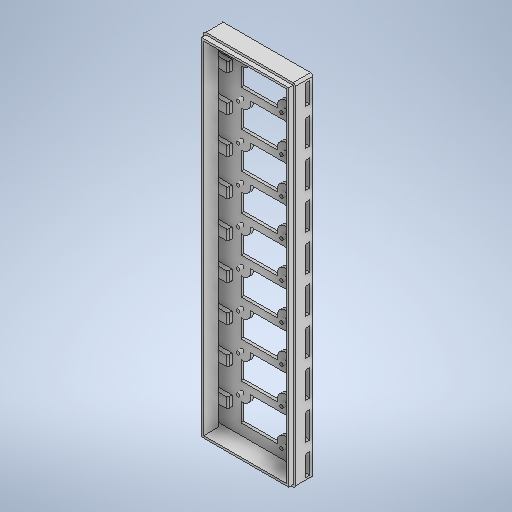
# Autodesk Inventor part: lm2596_socket
Saved by Autodesk Inventor 2025 (Build 290162000, 162)
## iProperties
Created: 2025-01-25
Part Number: lm2596_socket
Material: Všeobecné
Document SubType Name: Modeling
Designer: lukas
Density: 1 g/cm^3
Appearance: Výchozí
Author: lukas
## iProperties of the stored document lm2596_socket_3D tisk.ipt
Created: 2025-01-25
Part Number: lm2596_socket_3D tisk
Material: Všeobecné
Document SubType Name: Modeling
Designer: lukas
Density: 1 g/cm^3
Appearance: Výchozí
Author: lukas
Autodesk Inventor part; units mm, degrees
ref_plane "YZ Plane" through (0, 0, 0) normal (1, 0, 0) x (0, 1, 0)
ref_plane "XZ Plane" through (0, 0, 0) normal (0, 1, 0) x (-1, 0, 0)
ref_plane "XY Plane" through (0, 0, 0) normal (0, 0, 1) x (1, 0, 0)
sketch "Náčrt1" plane through (0, 0, 0) normal (0, 0, 1) x (1, 0, 0)
  line L0 (0, 17.5) -> (0, -17.5) projected
  line L1 (-32.9, 0) -> (32.9, 0) projected
  line L2 (23.5, -12.5) -> (-23.5, -12.5)
  line L3 (-23.5, -12.5) -> (-23.5, 12.5)
  line L4 (-23.5, 12.5) -> (23.5, 12.5)
  line L5 (23.5, 12.5) -> (23.5, -12.5)
  point P0 (0, 0)
  dimension "d0" = 47
  dimension "d1" = 25
  constraints: 8 end point, 2 parallel, 1 horizontal, 1 perpendicular, 2 other
  measures "d0" distance between parallel lines of L3 L5
  measures "d1" distance between parallel lines of L4 L2
extrude "Vysunutí1" add sketch "Náčrt1" along normal blind 2
sketch "Náčrt2" plane through (0, 0, 2) normal (0, 0, 1) x (1, 0, 0)
  line L0 (23.5, 12.5) -> (-23.5, 12.5) projected
  line L1 (-23.5, 12.5) -> (-23.5, -12.5) projected
  line L2 (-23.5, -12.5) -> (23.5, -12.5) projected
  line L3 (23.5, -12.5) -> (23.5, 12.5) projected
  line L4 (0, 17.5) -> (0, -17.5) projected
  line L5 (-32.9, 0) -> (32.9, 0) projected
  circle A0 centre (-15, 8.5) radius 1.2
  circle A1 centre (15, -8.5) radius 1.2
  point P0 (0, 0)
  dimension "d4" = 2.4
  dimension "d5" = 4
  dimension "d9" = 180
  dimension "d18" = 8.5
  constraints: 2 centre point, 3 other
  measures "d4" diameter of A0
  measures "d5" distance from line of A0.centre L0
  measures "d18" distance from line of L1 A0.centre
extrude "Vysunutí2" add sketch "Náčrt2" along normal blind 3 contours A0 | A1
sketch "Náčrt3" plane through (0, 0, 2) normal (0, 0, 1) x (1, 0, 0)
  circle A0 centre (15, -8.5) radius 1.2 projected
  circle A1 centre (-15, 8.5) radius 1.2 projected
  line L0 (23.5, 12.5) -> (-23.5, 12.5) projected
  line L1 (-23.5, 12.5) -> (-23.5, -12.5) projected
  line L2 (-23.5, -12.5) -> (23.5, -12.5) projected
  line L3 (23.5, -12.5) -> (23.5, 12.5) projected
  line L4 (0, 17.5) -> (0, -17.5) projected
  line L5 (-32.9, 0) -> (32.9, 0) projected
  line L6 (-23.5, 12.5) -> (-23.5, -12.5) projected
  line L7 (-22, -3.5) -> (-23.5, -3.5)
  line L8 (-23.5, -3.5) -> (-23.5, 3.5)
  line L9 (-23.5, 3.5) -> (-22, 3.5)
  line L10 (-22, 3.5) -> (-22, -3.5)
  line L11 (23.5, -3.5) -> (22, -3.5)
  line L12 (22, -3.5) -> (22, 3.5)
  line L13 (22, 3.5) -> (23.5, 3.5)
  line L14 (23.5, 3.5) -> (23.5, -3.5)
  line L15 (22, -3.5) -> (23.5, -3.5)
  line L16 (23.5, -3.5) -> (23.5, 0)
  line L17 (23.5, 0) -> (22, 0)
  line L18 (22, 0) -> (22, -3.5)
  line L19 (-22, -3.5) -> (-23.5, -3.5)
  line L20 (-23.5, -3.5) -> (-23.5, 0)
  line L21 (-23.5, 0) -> (-22, 0)
  line L22 (-22, 0) -> (-22, -3.5)
  point P0 (0, 0)
  point P1 (22, 0)
  point P2 (-22, 0)
  point P3 (-23.5, 3.5)
  point P4 (-23.5, -3.5)
  dimension "d13" = 7
  dimension "d14" = 7
  dimension "d15" = 44
  constraints: 32 end point, 8 parallel, 4 horizontal, 4 perpendicular, 2 midpoint, 2 point on line, 3 other
  measures "d13" distance of L9.end L7.start
  measures "d14" distance of L11.end L12.end
  measures "d15" distance between parallel lines of L10 L12
extrude "Vysunutí3" add sketch "Náčrt3" along normal blind 3 contours L3 L5 L12 L13 | L3 L11 L12 L5 | L9 L10 L5 L1 | L10 L7 L1 L5
sketch "Náčrt4" plane through (0, 0, 2) normal (0, 0, 1) x (1, 0, 0)
  line L0 (22, 3.5) -> (23.5, 3.5) projected
  line L1 (23.5, 3.5) -> (23.5, 12.5) projected
  line L2 (23.5, 12.5) -> (-23.5, 12.5) projected
  line L3 (-23.5, 12.5) -> (-23.5, 3.5) projected
  line L4 (-23.5, 3.5) -> (-22, 3.5) projected
  line L5 (-22, 3.5) -> (-22, -3.5) projected
  line L6 (-22, -3.5) -> (-23.5, -3.5) projected
  line L7 (-23.5, -3.5) -> (-23.5, -12.5) projected
  line L8 (-23.5, -12.5) -> (23.5, -12.5) projected
  line L9 (23.5, -12.5) -> (23.5, -3.5) projected
  line L10 (23.5, -3.5) -> (22, -3.5) projected
  line L11 (22, -3.5) -> (22, 3.5) projected
  circle A0 centre (15, -8.5) radius 1.2 projected
  circle A1 centre (-15, 8.5) radius 1.2 projected
  line L12 (15.8095, 10) -> (15.8095, -2.5549)
  line L13 (-15.8095, -10) -> (-15.8095, 2.5549)
  line L14 (0, 17.5) -> (0, -17.5) projected
  line L15 (-32.9, 0) -> (32.9, 0) projected
  arc A2 (-15.8095, 2.5549) -> (-9.1905, 10) centre (-15, 8.5) ccw
  arc A3 (15.8095, -2.5549) -> (9.1905, -10) centre (15, -8.5) ccw
  line L16 (-9.1905, 10) -> (15.8095, 10)
  line L17 (9.1905, -10) -> (-15.8095, -10)
  point P0 (0, 0)
  dimension "d21" = 12
  dimension "d22" = 12
  dimension "d23" = 20
  dimension "d25" = 25
  dimension "d26" = 25
  constraints: 8 end point, 4 point on circle, 2 centre point, 2 coincident, 2 parallel, 1 horizontal, 1 perpendicular, 1 other
  measures "d21" diameter of A2
  measures "d22" diameter of A3
  measures "d23" distance between parallel lines of L16 L17
  measures "d25" distance of L16.start L12.start
  measures "d26" distance of L17.start L13.start
extrude "Vysunutí4" cut sketch "Náčrt4" against normal through all contours L15 L14 L16 L12 | L12 A3 L17 L14 L15 | L15 L13 A2 L16 L14 | L14 L17 L13 L15
pattern_linear "Obdélníkové pole1" count 9 spacing 25 along (0, 1, 0) first direction both ways yes
sketch "Náčrt5" plane through (0, 0, 0) normal (0, 0, 1) x (1, 0, 0)
  line L0 (-15.8095, 15) -> (9.1905, 15) projected
  arc A0 (15.8095, 22.4451) -> (9.1905, 15) centre (15, 16.5) ccw projected
  line L1 (15.8095, 22.4451) -> (15.8095, 35) projected
  line L2 (15.8095, 35) -> (-9.1905, 35) projected
  arc A1 (-15.8095, 27.5549) -> (-9.1905, 35) centre (-15, 33.5) ccw projected
  line L3 (-15.8095, 27.5549) -> (-15.8095, 15) projected
  line L4 (-15.8095, 40) -> (9.1905, 40) projected
  arc A2 (15.8095, 47.4451) -> (9.1905, 40) centre (15, 41.5) ccw projected
  line L5 (15.8095, 47.4451) -> (15.8095, 60) projected
  line L6 (15.8095, 60) -> (-9.1905, 60) projected
  arc A3 (-15.8095, 52.5549) -> (-9.1905, 60) centre (-15, 58.5) ccw projected
  line L7 (-15.8095, 52.5549) -> (-15.8095, 40) projected
  line L8 (-15.8095, 65) -> (9.1905, 65) projected
  arc A4 (15.8095, 72.4451) -> (9.1905, 65) centre (15, 66.5) ccw projected
  line L9 (15.8095, 72.4451) -> (15.8095, 85) projected
  line L10 (15.8095, 85) -> (-9.1905, 85) projected
  arc A5 (-15.8095, 77.5549) -> (-9.1905, 85) centre (-15, 83.5) ccw projected
  line L11 (-15.8095, 77.5549) -> (-15.8095, 65) projected
  line L12 (-15.8095, 90) -> (9.1905, 90) projected
  arc A6 (15.8095, 97.4451) -> (9.1905, 90) centre (15, 91.5) ccw projected
  line L13 (15.8095, 97.4451) -> (15.8095, 110) projected
  line L14 (15.8095, 110) -> (-9.1905, 110) projected
  arc A7 (-15.8095, 102.5549) -> (-9.1905, 110) centre (-15, 108.5) ccw projected
  line L15 (-15.8095, 102.5549) -> (-15.8095, 90) projected
  line L16 (-15.8095, -110) -> (9.1905, -110) projected
  arc A8 (15.8095, -102.5549) -> (9.1905, -110) centre (15, -108.5) ccw projected
  line L17 (15.8095, -102.5549) -> (15.8095, -90) projected
  line L18 (15.8095, -90) -> (-9.1905, -90) projected
  arc A9 (-15.8095, -97.4451) -> (-9.1905, -90) centre (-15, -91.5) ccw projected
  line L19 (-15.8095, -97.4451) -> (-15.8095, -110) projected
  line L20 (-15.8095, -85) -> (9.1905, -85) projected
  arc A10 (15.8095, -77.5549) -> (9.1905, -85) centre (15, -83.5) ccw projected
  line L21 (15.8095, -77.5549) -> (15.8095, -65) projected
  line L22 (15.8095, -65) -> (-9.1905, -65) projected
  arc A11 (-15.8095, -72.4451) -> (-9.1905, -65) centre (-15, -66.5) ccw projected
  line L23 (-15.8095, -72.4451) -> (-15.8095, -85) projected
  line L24 (-15.8095, -60) -> (9.1905, -60) projected
  arc A12 (15.8095, -52.5549) -> (9.1905, -60) centre (15, -58.5) ccw projected
  line L25 (15.8095, -52.5549) -> (15.8095, -40) projected
  line L26 (15.8095, -40) -> (-9.1905, -40) projected
  arc A13 (-15.8095, -47.4451) -> (-9.1905, -40) centre (-15, -41.5) ccw projected
  line L27 (-15.8095, -47.4451) -> (-15.8095, -60) projected
  line L28 (-15.8095, -35) -> (9.1905, -35) projected
  arc A14 (15.8095, -27.5549) -> (9.1905, -35) centre (15, -33.5) ccw projected
  line L29 (15.8095, -27.5549) -> (15.8095, -15) projected
  line L30 (15.8095, -15) -> (-9.1905, -15) projected
  arc A15 (-15.8095, -22.4451) -> (-9.1905, -15) centre (-15, -16.5) ccw projected
  line L31 (-15.8095, -22.4451) -> (-15.8095, -35) projected
  line L32 (-15.8095, -10) -> (9.1905, -10) projected
  arc A16 (15.8095, -2.5549) -> (9.1905, -10) centre (15, -8.5) ccw projected
  line L33 (15.8095, -2.5549) -> (15.8095, 10) projected
  line L34 (15.8095, 10) -> (-9.1905, 10) projected
  arc A17 (-15.8095, 2.5549) -> (-9.1905, 10) centre (-15, 8.5) ccw projected
  line L35 (-15.8095, 2.5549) -> (-15.8095, -10) projected
  line L36 (23.5, -112.5) -> (23.5, 112.5) projected
  line L37 (-23.5, -112.5) -> (23.5, -112.5) projected
  line L38 (-23.5, 112.5) -> (-23.5, -112.5) projected
  line L39 (23.5, 112.5) -> (-23.5, 112.5) projected
  line L40 (31.5, 120.5) -> (31.5, -120.5)
  line L41 (31.5, -120.5) -> (-31.5, -120.5)
  line L42 (-31.5, -120.5) -> (-31.5, 120.5)
  line L43 (-31.5, 120.5) -> (31.5, 120.5)
  line L44 (23.5, 112.5) -> (-23.5, 112.5)
  line L45 (-23.5, 112.5) -> (-23.5, -112.5)
  line L46 (-23.5, -112.5) -> (23.5, -112.5)
  line L47 (23.5, -112.5) -> (23.5, 112.5)
  point P0 (0, 0)
  dimension "d33" = 8
  constraints: 16 end point, 2 parallel, 1 horizontal, 1 perpendicular, 3 other
  measures "d33" distance between parallel lines of L36 L40
extrude "Vysunutí5" add sketch "Náčrt5" along normal blind 2 contours L40 L41 L42 L43
sketch "Náčrt6" plane through (0, 0, 2) normal (0, 0, 1) x (1, 0, 0)
  line L0 (-23.5, -21.5) -> (-22, -21.5) projected
  line L1 (-22, -21.5) -> (-22, -28.5) projected
  line L2 (-22, -28.5) -> (-23.5, -28.5) projected
  line L3 (-23.5, -21.5) -> (-23.5, -28.5) projected
  line L4 (-23.5, -46.5) -> (-22, -46.5) projected
  line L5 (-22, -46.5) -> (-22, -53.5) projected
  line L6 (-22, -53.5) -> (-23.5, -53.5) projected
  line L7 (-23.5, -46.5) -> (-23.5, -53.5) projected
  line L8 (-23.5, 3.5) -> (-23.5, -3.5) projected
  line L9 (-23.5, 3.5) -> (-22, 3.5) projected
  line L10 (-22, 3.5) -> (-22, -3.5) projected
  line L11 (-22, -3.5) -> (-23.5, -3.5) projected
  line L12 (-23.5, -71.5) -> (-22, -71.5) projected
  line L13 (-22, -71.5) -> (-22, -78.5) projected
  line L14 (-22, -78.5) -> (-23.5, -78.5) projected
  line L15 (-23.5, -71.5) -> (-23.5, -78.5) projected
  line L16 (23.5, -28.5) -> (22, -28.5) projected
  line L17 (22, -28.5) -> (22, -21.5) projected
  line L18 (22, -21.5) -> (23.5, -21.5) projected
  line L19 (23.5, -28.5) -> (23.5, -21.5) projected
  line L20 (23.5, -53.5) -> (23.5, -46.5) projected
  line L21 (23.5, -53.5) -> (22, -53.5) projected
  line L22 (22, -53.5) -> (22, -46.5) projected
  line L23 (22, -46.5) -> (23.5, -46.5) projected
  line L24 (-23.5, 28.5) -> (-23.5, 21.5) projected
  line L25 (-23.5, 28.5) -> (-22, 28.5) projected
  line L26 (-22, 28.5) -> (-22, 21.5) projected
  line L27 (-22, 21.5) -> (-23.5, 21.5) projected
  line L28 (-23.5, -96.5) -> (-22, -96.5) projected
  line L29 (-22, -96.5) -> (-22, -103.5) projected
  line L30 (-22, -103.5) -> (-23.5, -103.5) projected
  line L31 (-23.5, -96.5) -> (-23.5, -103.5) projected
  line L32 (23.5, -3.5) -> (22, -3.5) projected
  line L33 (22, -3.5) -> (22, 3.5) projected
  line L34 (22, 3.5) -> (23.5, 3.5) projected
  line L35 (23.5, -3.5) -> (23.5, 3.5) projected
  line L36 (23.5, -78.5) -> (23.5, -71.5) projected
  line L37 (23.5, -78.5) -> (22, -78.5) projected
  line L38 (22, -78.5) -> (22, -71.5) projected
  line L39 (22, -71.5) -> (23.5, -71.5) projected
  line L40 (-23.5, 53.5) -> (-23.5, 46.5) projected
  line L41 (-23.5, 53.5) -> (-22, 53.5) projected
  line L42 (-22, 53.5) -> (-22, 46.5) projected
  line L43 (-22, 46.5) -> (-23.5, 46.5) projected
  line L44 (23.5, 21.5) -> (22, 21.5) projected
  line L45 (22, 21.5) -> (22, 28.5) projected
  line L46 (22, 28.5) -> (23.5, 28.5) projected
  line L47 (23.5, 21.5) -> (23.5, 28.5) projected
  line L48 (23.5, -103.5) -> (23.5, -96.5) projected
  line L49 (23.5, -103.5) -> (22, -103.5) projected
  line L50 (22, -103.5) -> (22, -96.5) projected
  line L51 (22, -96.5) -> (23.5, -96.5) projected
  line L52 (-23.5, 78.5) -> (-23.5, 71.5) projected
  line L53 (-23.5, 78.5) -> (-22, 78.5) projected
  line L54 (-22, 78.5) -> (-22, 71.5) projected
  line L55 (-22, 71.5) -> (-23.5, 71.5) projected
  line L56 (23.5, 46.5) -> (22, 46.5) projected
  line L57 (22, 46.5) -> (22, 53.5) projected
  line L58 (22, 53.5) -> (23.5, 53.5) projected
  line L59 (23.5, 46.5) -> (23.5, 53.5) projected
  line L60 (23.5, 71.5) -> (22, 71.5) projected
  line L61 (22, 71.5) -> (22, 78.5) projected
  line L62 (22, 78.5) -> (23.5, 78.5) projected
  line L63 (23.5, 71.5) -> (23.5, 78.5) projected
  line L64 (-23.5, 103.5) -> (-23.5, 96.5) projected
  line L65 (-23.5, 103.5) -> (-22, 103.5) projected
  line L66 (-22, 103.5) -> (-22, 96.5) projected
  line L67 (-22, 96.5) -> (-23.5, 96.5) projected
  line L68 (-31.5, 120.5) -> (-31.5, -120.5) projected
  line L69 (-31.5, -120.5) -> (31.5, -120.5) projected
  line L70 (31.5, -120.5) -> (31.5, 120.5) projected
  line L71 (31.5, 120.5) -> (-31.5, 120.5) projected
  circle A0 centre (-15, 33.5) radius 1.2 projected
  circle A1 centre (15, 16.5) radius 1.2 projected
  line L72 (9.1905, 15) -> (-15.8095, 15) projected
  line L73 (-15.8095, 15) -> (-15.8095, 27.5549) projected
  arc A2 (-15.8095, 27.5549) -> (-9.1905, 35) centre (-15, 33.5) ccw projected
  line L74 (-9.1905, 35) -> (15.8095, 35) projected
  line L75 (15.8095, 35) -> (15.8095, 22.4451) projected
  arc A3 (15.8095, 22.4451) -> (9.1905, 15) centre (15, 16.5) ccw projected
  line L76 (9.1905, 40) -> (-15.8095, 40) projected
  line L77 (-15.8095, 40) -> (-15.8095, 52.5549) projected
  arc A4 (-15.8095, 52.5549) -> (-9.1905, 60) centre (-15, 58.5) ccw projected
  line L78 (-9.1905, 60) -> (15.8095, 60) projected
  line L79 (15.8095, 60) -> (15.8095, 47.4451) projected
  arc A5 (15.8095, 47.4451) -> (9.1905, 40) centre (15, 41.5) ccw projected
  circle A6 centre (15, 41.5) radius 1.2 projected
  circle A7 centre (-15, 58.5) radius 1.2 projected
  line L80 (9.1905, 65) -> (-15.8095, 65) projected
  line L81 (-15.8095, 65) -> (-15.8095, 77.5549) projected
  arc A8 (-15.8095, 77.5549) -> (-9.1905, 85) centre (-15, 83.5) ccw projected
  line L82 (-9.1905, 85) -> (15.8095, 85) projected
  line L83 (15.8095, 85) -> (15.8095, 72.4451) projected
  arc A9 (15.8095, 72.4451) -> (9.1905, 65) centre (15, 66.5) ccw projected
  circle A10 centre (15, 66.5) radius 1.2 projected
  circle A11 centre (-15, 83.5) radius 1.2 projected
  line L84 (9.1905, 90) -> (-15.8095, 90) projected
  line L85 (-15.8095, 90) -> (-15.8095, 102.5549) projected
  arc A12 (-15.8095, 102.5549) -> (-9.1905, 110) centre (-15, 108.5) ccw projected
  line L86 (-9.1905, 110) -> (15.8095, 110) projected
  line L87 (15.8095, 110) -> (15.8095, 97.4451) projected
  arc A13 (15.8095, 97.4451) -> (9.1905, 90) centre (15, 91.5) ccw projected
  circle A14 centre (15, 91.5) radius 1.2 projected
  circle A15 centre (-15, 108.5) radius 1.2 projected
  circle A16 centre (-15, -91.5) radius 1.2 projected
  circle A17 centre (15, -108.5) radius 1.2 projected
  line L88 (9.1905, -110) -> (-15.8095, -110) projected
  line L89 (-15.8095, -110) -> (-15.8095, -97.4451) projected
  arc A18 (-15.8095, -97.4451) -> (-9.1905, -90) centre (-15, -91.5) ccw projected
  line L90 (-9.1905, -90) -> (15.8095, -90) projected
  line L91 (15.8095, -90) -> (15.8095, -102.5549) projected
  arc A19 (15.8095, -102.5549) -> (9.1905, -110) centre (15, -108.5) ccw projected
  line L92 (9.1905, -85) -> (-15.8095, -85) projected
  line L93 (-15.8095, -85) -> (-15.8095, -72.4451) projected
  arc A20 (-15.8095, -72.4451) -> (-9.1905, -65) centre (-15, -66.5) ccw projected
  line L94 (-9.1905, -65) -> (15.8095, -65) projected
  line L95 (15.8095, -65) -> (15.8095, -77.5549) projected
  arc A21 (15.8095, -77.5549) -> (9.1905, -85) centre (15, -83.5) ccw projected
  circle A22 centre (15, -83.5) radius 1.2 projected
  circle A23 centre (-15, -66.5) radius 1.2 projected
  line L96 (9.1905, -60) -> (-15.8095, -60) projected
  line L97 (-15.8095, -60) -> (-15.8095, -47.4451) projected
  arc A24 (-15.8095, -47.4451) -> (-9.1905, -40) centre (-15, -41.5) ccw projected
  line L98 (-9.1905, -40) -> (15.8095, -40) projected
  line L99 (15.8095, -40) -> (15.8095, -52.5549) projected
  arc A25 (15.8095, -52.5549) -> (9.1905, -60) centre (15, -58.5) ccw projected
  circle A26 centre (15, -58.5) radius 1.2 projected
  circle A27 centre (-15, -41.5) radius 1.2 projected
  line L100 (9.1905, -35) -> (-15.8095, -35) projected
  line L101 (-15.8095, -35) -> (-15.8095, -22.4451) projected
  arc A28 (-15.8095, -22.4451) -> (-9.1905, -15) centre (-15, -16.5) ccw projected
  line L102 (-9.1905, -15) -> (15.8095, -15) projected
  line L103 (15.8095, -15) -> (15.8095, -27.5549) projected
  arc A29 (15.8095, -27.5549) -> (9.1905, -35) centre (15, -33.5) ccw projected
  circle A30 centre (15, -33.5) radius 1.2 projected
  circle A31 centre (-15, -16.5) radius 1.2 projected
  line L104 (9.1905, -10) -> (-15.8095, -10) projected
  line L105 (-15.8095, -10) -> (-15.8095, 2.5549) projected
  arc A32 (-15.8095, 2.5549) -> (-9.1905, 10) centre (-15, 8.5) ccw projected
  line L106 (-9.1905, 10) -> (15.8095, 10) projected
  line L107 (15.8095, 10) -> (15.8095, -2.5549) projected
  arc A33 (15.8095, -2.5549) -> (9.1905, -10) centre (15, -8.5) ccw projected
  line L108 (23.5, 96.5) -> (23.5, 103.5) projected
  line L109 (23.5, 96.5) -> (22, 96.5) projected
  line L110 (22, 96.5) -> (22, 103.5) projected
  line L111 (22, 103.5) -> (23.5, 103.5) projected
  circle A34 centre (15, -8.5) radius 1.2 projected
  circle A35 centre (-15, 8.5) radius 1.2 projected
  line L112 (28.5, 117.5) -> (28.5, -117.5)
  line L113 (28.5, -117.5) -> (-28.5, -117.5)
  line L114 (-28.5, -117.5) -> (-28.5, 117.5)
  line L115 (-28.5, 117.5) -> (28.5, 117.5)
  line L116 (31.5, 120.5) -> (-31.5, 120.5)
  line L117 (-31.5, 120.5) -> (-31.5, -120.5)
  line L118 (-31.5, -120.5) -> (31.5, -120.5)
  line L119 (31.5, -120.5) -> (31.5, 120.5)
  point P0 (0, 0)
  dimension "d36" = 3
  constraints: 16 end point, 2 parallel, 1 horizontal, 1 perpendicular, 3 other
  measures "d36" distance between parallel lines of L70 L112
extrude "Vysunutí6" add sketch "Náčrt6" along normal blind 10 contours L71 L70 L69 L68
sketch "Náčrt7" plane through (-31.5, -120.5, 0) normal (-1, 0, 0) x (0, 0, 1)
  line L0 (0, 289.2) -> (0, -48.2) projected
  line L1 (-2.4, 120.5) -> (14.4, 120.5) projected
  line L2 (2, 238) -> (2, 3) projected
  line L3 (2, 3) -> (2, 238) projected
  line L4 (2, 99) -> (2, 92) projected
  line L5 (2, 99) -> (2, 92) projected
  line L6 (2, 74) -> (2, 67) projected
  line L7 (2, 74) -> (2, 67) projected
  line L8 (2, 124) -> (2, 117) projected
  line L9 (2, 124) -> (2, 117) projected
  line L10 (2, 49) -> (2, 42) projected
  line L11 (2, 49) -> (2, 42) projected
  line L12 (2, 92) -> (2, 99) projected
  line L13 (2, 92) -> (2, 99) projected
  line L14 (2, 67) -> (2, 74) projected
  line L15 (2, 67) -> (2, 74) projected
  line L16 (2, 149) -> (2, 142) projected
  line L17 (2, 149) -> (2, 142) projected
  line L18 (2, 24) -> (2, 17) projected
  line L19 (2, 24) -> (2, 17) projected
  line L20 (2, 117) -> (2, 124) projected
  line L21 (2, 117) -> (2, 124) projected
  line L22 (2, 42) -> (2, 49) projected
  line L23 (2, 42) -> (2, 49) projected
  line L24 (2, 174) -> (2, 167) projected
  line L25 (2, 174) -> (2, 167) projected
  line L26 (2, 142) -> (2, 149) projected
  line L27 (2, 142) -> (2, 149) projected
  line L28 (2, 17) -> (2, 24) projected
  line L29 (2, 17) -> (2, 24) projected
  line L30 (2, 199) -> (2, 192) projected
  line L31 (2, 199) -> (2, 192) projected
  line L32 (2, 167) -> (2, 174) projected
  line L33 (2, 167) -> (2, 174) projected
  line L34 (2, 192) -> (2, 199) projected
  line L35 (2, 192) -> (2, 199) projected
  line L36 (2, 224) -> (2, 217) projected
  line L37 (2, 224) -> (2, 217) projected
  line L38 (2, 155.2) -> (2, 152.8) projected
  line L39 (2, 138.2) -> (2, 135.8) projected
  line L40 (2, 135.5) -> (2, 148.0549) projected
  line L41 (2, 148.0549) -> (2, 155.5) projected
  line L42 (2, 155.5) -> (2, 142.9451) projected
  line L43 (2, 142.9451) -> (2, 135.5) projected
  line L44 (2, 160.5) -> (2, 173.0549) projected
  line L45 (2, 173.0549) -> (2, 180.5) projected
  line L46 (2, 180.5) -> (2, 167.9451) projected
  line L47 (2, 167.9451) -> (2, 160.5) projected
  line L48 (2, 163.2) -> (2, 160.8) projected
  line L49 (2, 180.2) -> (2, 177.8) projected
  line L50 (2, 185.5) -> (2, 198.0549) projected
  line L51 (2, 198.0549) -> (2, 205.5) projected
  line L52 (2, 205.5) -> (2, 192.9451) projected
  line L53 (2, 192.9451) -> (2, 185.5) projected
  line L54 (2, 188.2) -> (2, 185.8) projected
  line L55 (2, 205.2) -> (2, 202.8) projected
  line L56 (2, 210.5) -> (2, 223.0549) projected
  line L57 (2, 223.0549) -> (2, 230.5) projected
  line L58 (2, 230.5) -> (2, 217.9451) projected
  line L59 (2, 217.9451) -> (2, 210.5) projected
  line L60 (2, 213.2) -> (2, 210.8) projected
  line L61 (2, 230.2) -> (2, 227.8) projected
  line L62 (2, 30.2) -> (2, 27.8) projected
  line L63 (2, 13.2) -> (2, 10.8) projected
  line L64 (2, 10.5) -> (2, 23.0549) projected
  line L65 (2, 23.0549) -> (2, 30.5) projected
  line L66 (2, 30.5) -> (2, 17.9451) projected
  line L67 (2, 17.9451) -> (2, 10.5) projected
  line L68 (2, 35.5) -> (2, 48.0549) projected
  line L69 (2, 48.0549) -> (2, 55.5) projected
  line L70 (2, 55.5) -> (2, 42.9451) projected
  line L71 (2, 42.9451) -> (2, 35.5) projected
  line L72 (2, 38.2) -> (2, 35.8) projected
  line L73 (2, 55.2) -> (2, 52.8) projected
  line L74 (2, 60.5) -> (2, 73.0549) projected
  line L75 (2, 73.0549) -> (2, 80.5) projected
  line L76 (2, 80.5) -> (2, 67.9451) projected
  line L77 (2, 67.9451) -> (2, 60.5) projected
  line L78 (2, 63.2) -> (2, 60.8) projected
  line L79 (2, 80.2) -> (2, 77.8) projected
  line L80 (2, 85.5) -> (2, 98.0549) projected
  line L81 (2, 98.0549) -> (2, 105.5) projected
  line L82 (2, 105.5) -> (2, 92.9451) projected
  line L83 (2, 92.9451) -> (2, 85.5) projected
  line L84 (2, 88.2) -> (2, 85.8) projected
  line L85 (2, 105.2) -> (2, 102.8) projected
  line L86 (2, 110.5) -> (2, 123.0549) projected
  line L87 (2, 123.0549) -> (2, 130.5) projected
  line L88 (2, 130.5) -> (2, 117.9451) projected
  line L89 (2, 117.9451) -> (2, 110.5) projected
  line L90 (2, 217) -> (2, 224) projected
  line L91 (2, 217) -> (2, 224) projected
  line L92 (2, 113.2) -> (2, 110.8) projected
  line L93 (2, 130.2) -> (2, 127.8) projected
  line L94 (2, 238) -> (2, 3) projected
  line L95 (2, 238) -> (12, 238) projected
  line L96 (12, 3) -> (12, 238) projected
  line L97 (2, 3) -> (12, 3) projected
  line L98 (5, 224) -> (5, 217) projected
  line L99 (5, 217) -> (5, 224) projected
  line L100 (2, 3) -> (2, 238) projected
  line L101 (5, 238) -> (2, 238)
  line L102 (2, 238) -> (2, 3)
  line L103 (2, 3) -> (5, 3)
  line L104 (5, 3) -> (5, 238)
  point P0 (0, 120.5)
  point P1 (2, 3)
  point P2 (5, 3)
  constraints: 8 end point, 2 parallel, 2 point on line, 1 horizontal, 1 perpendicular
extrude "Vysunutí7" cut sketch "Náčrt7" against normal up to surface (3 mm away) contours L2 L95 L104 L98 L1 | L1 L104 L97 L2
sketch "Náčrt8" plane through (0, 0, 2) normal (0, 0, 1) x (1, 0, 0)
  line L0 (28.5, 117.5) -> (-31.5, 117.5) projected
  line L1 (-31.5, -117.5) -> (-31.5, 117.5) projected
  line L2 (-31.5, -117.5) -> (28.5, -117.5) projected
  line L3 (28.5, -117.5) -> (28.5, 117.5) projected
  line L4 (-23.5, -21.5) -> (-22, -21.5) projected
  line L5 (-22, -21.5) -> (-22, -28.5) projected
  line L6 (-22, -28.5) -> (-23.5, -28.5) projected
  line L7 (-23.5, -21.5) -> (-23.5, -28.5) projected
  line L8 (-23.5, -46.5) -> (-22, -46.5) projected
  line L9 (-22, -46.5) -> (-22, -53.5) projected
  line L10 (-22, -53.5) -> (-23.5, -53.5) projected
  line L11 (-23.5, -46.5) -> (-23.5, -53.5) projected
  line L12 (-23.5, 3.5) -> (-23.5, -3.5) projected
  line L13 (-23.5, 3.5) -> (-22, 3.5) projected
  line L14 (-22, 3.5) -> (-22, -3.5) projected
  line L15 (-22, -3.5) -> (-23.5, -3.5) projected
  line L16 (-23.5, -71.5) -> (-22, -71.5) projected
  line L17 (-22, -71.5) -> (-22, -78.5) projected
  line L18 (-22, -78.5) -> (-23.5, -78.5) projected
  line L19 (-23.5, -71.5) -> (-23.5, -78.5) projected
  line L20 (23.5, -28.5) -> (22, -28.5) projected
  line L21 (22, -28.5) -> (22, -21.5) projected
  line L22 (22, -21.5) -> (23.5, -21.5) projected
  line L23 (23.5, -28.5) -> (23.5, -21.5) projected
  line L24 (23.5, -53.5) -> (23.5, -46.5) projected
  line L25 (23.5, -53.5) -> (22, -53.5) projected
  line L26 (22, -53.5) -> (22, -46.5) projected
  line L27 (22, -46.5) -> (23.5, -46.5) projected
  line L28 (-23.5, 28.5) -> (-23.5, 21.5) projected
  line L29 (-23.5, 28.5) -> (-22, 28.5) projected
  line L30 (-22, 28.5) -> (-22, 21.5) projected
  line L31 (-22, 21.5) -> (-23.5, 21.5) projected
  line L32 (-23.5, -96.5) -> (-22, -96.5) projected
  line L33 (-22, -96.5) -> (-22, -103.5) projected
  line L34 (-22, -103.5) -> (-23.5, -103.5) projected
  line L35 (-23.5, -96.5) -> (-23.5, -103.5) projected
  line L36 (23.5, -3.5) -> (22, -3.5) projected
  line L37 (22, -3.5) -> (22, 3.5) projected
  line L38 (22, 3.5) -> (23.5, 3.5) projected
  line L39 (23.5, -3.5) -> (23.5, 3.5) projected
  line L40 (23.5, -78.5) -> (23.5, -71.5) projected
  line L41 (23.5, -78.5) -> (22, -78.5) projected
  line L42 (22, -78.5) -> (22, -71.5) projected
  line L43 (22, -71.5) -> (23.5, -71.5) projected
  line L44 (-23.5, 53.5) -> (-23.5, 46.5) projected
  line L45 (-23.5, 53.5) -> (-22, 53.5) projected
  line L46 (-22, 53.5) -> (-22, 46.5) projected
  line L47 (-22, 46.5) -> (-23.5, 46.5) projected
  line L48 (23.5, 21.5) -> (22, 21.5) projected
  line L49 (22, 21.5) -> (22, 28.5) projected
  line L50 (22, 28.5) -> (23.5, 28.5) projected
  line L51 (23.5, 21.5) -> (23.5, 28.5) projected
  line L52 (23.5, -103.5) -> (23.5, -96.5) projected
  line L53 (23.5, -103.5) -> (22, -103.5) projected
  line L54 (22, -103.5) -> (22, -96.5) projected
  line L55 (22, -96.5) -> (23.5, -96.5) projected
  line L56 (-23.5, 78.5) -> (-23.5, 71.5) projected
  line L57 (-23.5, 78.5) -> (-22, 78.5) projected
  line L58 (-22, 78.5) -> (-22, 71.5) projected
  line L59 (-22, 71.5) -> (-23.5, 71.5) projected
  line L60 (23.5, 46.5) -> (22, 46.5) projected
  line L61 (22, 46.5) -> (22, 53.5) projected
  line L62 (22, 53.5) -> (23.5, 53.5) projected
  line L63 (23.5, 46.5) -> (23.5, 53.5) projected
  line L64 (23.5, 71.5) -> (22, 71.5) projected
  line L65 (22, 71.5) -> (22, 78.5) projected
  line L66 (22, 78.5) -> (23.5, 78.5) projected
  line L67 (23.5, 71.5) -> (23.5, 78.5) projected
  line L68 (-23.5, 103.5) -> (-23.5, 96.5) projected
  line L69 (-23.5, 103.5) -> (-22, 103.5) projected
  line L70 (-22, 103.5) -> (-22, 96.5) projected
  line L71 (-22, 96.5) -> (-23.5, 96.5) projected
  circle A0 centre (-15, 33.5) radius 1.2 projected
  circle A1 centre (15, 16.5) radius 1.2 projected
  line L72 (9.1905, 15) -> (-15.8095, 15) projected
  line L73 (-15.8095, 15) -> (-15.8095, 27.5549) projected
  arc A2 (-15.8095, 27.5549) -> (-9.1905, 35) centre (-15, 33.5) ccw projected
  line L74 (-9.1905, 35) -> (15.8095, 35) projected
  line L75 (15.8095, 35) -> (15.8095, 22.4451) projected
  arc A3 (15.8095, 22.4451) -> (9.1905, 15) centre (15, 16.5) ccw projected
  line L76 (9.1905, 40) -> (-15.8095, 40) projected
  line L77 (-15.8095, 40) -> (-15.8095, 52.5549) projected
  arc A4 (-15.8095, 52.5549) -> (-9.1905, 60) centre (-15, 58.5) ccw projected
  line L78 (-9.1905, 60) -> (15.8095, 60) projected
  line L79 (15.8095, 60) -> (15.8095, 47.4451) projected
  arc A5 (15.8095, 47.4451) -> (9.1905, 40) centre (15, 41.5) ccw projected
  circle A6 centre (15, 41.5) radius 1.2 projected
  circle A7 centre (-15, 58.5) radius 1.2 projected
  line L80 (9.1905, 65) -> (-15.8095, 65) projected
  line L81 (-15.8095, 65) -> (-15.8095, 77.5549) projected
  arc A8 (-15.8095, 77.5549) -> (-9.1905, 85) centre (-15, 83.5) ccw projected
  line L82 (-9.1905, 85) -> (15.8095, 85) projected
  line L83 (15.8095, 85) -> (15.8095, 72.4451) projected
  arc A9 (15.8095, 72.4451) -> (9.1905, 65) centre (15, 66.5) ccw projected
  circle A10 centre (15, 66.5) radius 1.2 projected
  circle A11 centre (-15, 83.5) radius 1.2 projected
  line L84 (9.1905, 90) -> (-15.8095, 90) projected
  line L85 (-15.8095, 90) -> (-15.8095, 102.5549) projected
  arc A12 (-15.8095, 102.5549) -> (-9.1905, 110) centre (-15, 108.5) ccw projected
  line L86 (-9.1905, 110) -> (15.8095, 110) projected
  line L87 (15.8095, 110) -> (15.8095, 97.4451) projected
  arc A13 (15.8095, 97.4451) -> (9.1905, 90) centre (15, 91.5) ccw projected
  circle A14 centre (15, 91.5) radius 1.2 projected
  circle A15 centre (-15, 108.5) radius 1.2 projected
  circle A16 centre (-15, -91.5) radius 1.2 projected
  circle A17 centre (15, -108.5) radius 1.2 projected
  line L88 (9.1905, -110) -> (-15.8095, -110) projected
  line L89 (-15.8095, -110) -> (-15.8095, -97.4451) projected
  arc A18 (-15.8095, -97.4451) -> (-9.1905, -90) centre (-15, -91.5) ccw projected
  line L90 (-9.1905, -90) -> (15.8095, -90) projected
  line L91 (15.8095, -90) -> (15.8095, -102.5549) projected
  arc A19 (15.8095, -102.5549) -> (9.1905, -110) centre (15, -108.5) ccw projected
  line L92 (9.1905, -85) -> (-15.8095, -85) projected
  line L93 (-15.8095, -85) -> (-15.8095, -72.4451) projected
  arc A20 (-15.8095, -72.4451) -> (-9.1905, -65) centre (-15, -66.5) ccw projected
  line L94 (-9.1905, -65) -> (15.8095, -65) projected
  line L95 (15.8095, -65) -> (15.8095, -77.5549) projected
  arc A21 (15.8095, -77.5549) -> (9.1905, -85) centre (15, -83.5) ccw projected
  circle A22 centre (15, -83.5) radius 1.2 projected
  circle A23 centre (-15, -66.5) radius 1.2 projected
  line L96 (9.1905, -60) -> (-15.8095, -60) projected
  line L97 (-15.8095, -60) -> (-15.8095, -47.4451) projected
  arc A24 (-15.8095, -47.4451) -> (-9.1905, -40) centre (-15, -41.5) ccw projected
  line L98 (-9.1905, -40) -> (15.8095, -40) projected
  line L99 (15.8095, -40) -> (15.8095, -52.5549) projected
  arc A25 (15.8095, -52.5549) -> (9.1905, -60) centre (15, -58.5) ccw projected
  circle A26 centre (15, -58.5) radius 1.2 projected
  circle A27 centre (-15, -41.5) radius 1.2 projected
  line L100 (9.1905, -35) -> (-15.8095, -35) projected
  line L101 (-15.8095, -35) -> (-15.8095, -22.4451) projected
  arc A28 (-15.8095, -22.4451) -> (-9.1905, -15) centre (-15, -16.5) ccw projected
  line L102 (-9.1905, -15) -> (15.8095, -15) projected
  line L103 (15.8095, -15) -> (15.8095, -27.5549) projected
  arc A29 (15.8095, -27.5549) -> (9.1905, -35) centre (15, -33.5) ccw projected
  circle A30 centre (15, -33.5) radius 1.2 projected
  circle A31 centre (-15, -16.5) radius 1.2 projected
  line L104 (9.1905, -10) -> (-15.8095, -10) projected
  line L105 (-15.8095, -10) -> (-15.8095, 2.5549) projected
  arc A32 (-15.8095, 2.5549) -> (-9.1905, 10) centre (-15, 8.5) ccw projected
  line L106 (-9.1905, 10) -> (15.8095, 10) projected
  line L107 (15.8095, 10) -> (15.8095, -2.5549) projected
  arc A33 (15.8095, -2.5549) -> (9.1905, -10) centre (15, -8.5) ccw projected
  line L108 (23.5, 96.5) -> (23.5, 103.5) projected
  line L109 (23.5, 96.5) -> (22, 96.5) projected
  line L110 (22, 96.5) -> (22, 103.5) projected
  line L111 (22, 103.5) -> (23.5, 103.5) projected
  circle A34 centre (15, -8.5) radius 1.2 projected
  circle A35 centre (-15, 8.5) radius 1.2 projected
  line L112 (-23.5, 3.5) -> (-31.5, 3.5)
  line L113 (-31.5, 3.5) -> (-31.5, -3.5)
  line L114 (-31.5, -3.5) -> (-23.5, -3.5)
  line L115 (-23.5, -3.5) -> (-23.5, 3.5)
  line L116 (-23.5, 28.5) -> (-31.5, 28.5)
  line L117 (-31.5, 28.5) -> (-31.5, 21.5)
  line L118 (-31.5, 21.5) -> (-23.5, 21.5)
  line L119 (-23.5, 21.5) -> (-23.5, 28.5)
  line L120 (-23.5, 53.5) -> (-31.5, 53.5)
  line L121 (-31.5, 53.5) -> (-31.5, 46.5)
  line L122 (-31.5, 46.5) -> (-23.5, 46.5)
  line L123 (-23.5, 46.5) -> (-23.5, 53.5)
  line L124 (-23.5, 78.5) -> (-31.5, 78.5)
  line L125 (-31.5, 78.5) -> (-31.5, 71.5)
  line L126 (-31.5, 71.5) -> (-23.5, 71.5)
  line L127 (-23.5, 71.5) -> (-23.5, 78.5)
  line L128 (-23.5, 103.5) -> (-23.5, 96.5) projected
  line L129 (-23.5, 103.5) -> (-31.5, 103.5)
  line L130 (-31.5, 103.5) -> (-31.5, 96.5)
  line L131 (-31.5, 96.5) -> (-23.5, 96.5)
  line L132 (-23.5, 96.5) -> (-23.5, 103.5)
  line L133 (-23.5, -21.5) -> (-31.5, -21.5)
  line L134 (-31.5, -21.5) -> (-31.5, -28.5)
  line L135 (-31.5, -28.5) -> (-23.5, -28.5)
  line L136 (-23.5, -28.5) -> (-23.5, -21.5)
  line L137 (-23.5, -46.5) -> (-31.5, -46.5)
  line L138 (-31.5, -46.5) -> (-31.5, -53.5)
  line L139 (-31.5, -53.5) -> (-23.5, -53.5)
  line L140 (-23.5, -53.5) -> (-23.5, -46.5)
  line L141 (-23.5, -71.5) -> (-31.5, -71.5)
  line L142 (-31.5, -71.5) -> (-31.5, -78.5)
  line L143 (-31.5, -78.5) -> (-23.5, -78.5)
  line L144 (-23.5, -78.5) -> (-23.5, -71.5)
  line L145 (-23.5, -96.5) -> (-31.5, -96.5)
  line L146 (-31.5, -96.5) -> (-31.5, -103.5)
  line L147 (-31.5, -103.5) -> (-23.5, -103.5)
  line L148 (-23.5, -103.5) -> (-23.5, -96.5)
  point P0 (0, 0)
  point P1 (-31.5, 3.5)
  point P2 (-31.5, 103.5)
  point P3 (-31.5, 78.5)
  point P4 (-31.5, 53.5)
  point P5 (-31.5, 28.5)
  point P6 (-31.5, -21.5)
  point P7 (-31.5, -96.5)
  point P8 (-31.5, -71.5)
  point P9 (-31.5, -46.5)
  constraints: 72 end point, 18 parallel, 9 horizontal, 9 perpendicular, 9 point on line, 10 other
extrude "Vysunutí8" add sketch "Náčrt8" along normal up to surface (3 mm away) contours L129 L68 L131 L1 | L1 L145 L35 L147 | L124 L56 L126 L1 | L1 L141 L19 L143 | L120 L44 L122 L1 | L1 L137 L11 L139 | L116 L28 L118 L1 | L1 L133 L7 L135 | L112 L12 L114 L1
sketch "Náčrt9" plane through (31.5, -120.5, 0) normal (1, 0, 0) x (0, 0, -1)
  line L0 (0, 0) -> (0, 241) projected
  line L1 (0, 241) -> (-12, 241) projected
  line L2 (-12, 0) -> (-12, 241) projected
  line L3 (0, 0) -> (-12, 0) projected
  line L4 (-2, 127.8) -> (-2, 130.2) projected
  line L5 (-2, 110.8) -> (-2, 113.2) projected
  line L6 (-2, 217) -> (-2, 224) projected
  line L7 (-2, 217) -> (-2, 224) projected
  line L8 (-2, 110.5) -> (-2, 123.0549) projected
  line L9 (-2, 123.0549) -> (-2, 130.5) projected
  line L10 (-2, 130.5) -> (-2, 117.9451) projected
  line L11 (-2, 117.9451) -> (-2, 110.5) projected
  line L12 (-2, 102.8) -> (-2, 105.2) projected
  line L13 (-2, 85.8) -> (-2, 88.2) projected
  line L14 (-2, 85.5) -> (-2, 98.0549) projected
  line L15 (-2, 98.0549) -> (-2, 105.5) projected
  line L16 (-2, 105.5) -> (-2, 92.9451) projected
  line L17 (-2, 92.9451) -> (-2, 85.5) projected
  line L18 (-2, 77.8) -> (-2, 80.2) projected
  line L19 (-2, 60.8) -> (-2, 63.2) projected
  line L20 (-2, 60.5) -> (-2, 73.0549) projected
  line L21 (-2, 73.0549) -> (-2, 80.5) projected
  line L22 (-2, 80.5) -> (-2, 67.9451) projected
  line L23 (-2, 67.9451) -> (-2, 60.5) projected
  line L24 (-2, 52.8) -> (-2, 55.2) projected
  line L25 (-2, 35.8) -> (-2, 38.2) projected
  line L26 (-2, 35.5) -> (-2, 48.0549) projected
  line L27 (-2, 48.0549) -> (-2, 55.5) projected
  line L28 (-2, 55.5) -> (-2, 42.9451) projected
  line L29 (-2, 42.9451) -> (-2, 35.5) projected
  line L30 (-2, 10.5) -> (-2, 23.0549) projected
  line L31 (-2, 23.0549) -> (-2, 30.5) projected
  line L32 (-2, 30.5) -> (-2, 17.9451) projected
  line L33 (-2, 17.9451) -> (-2, 10.5) projected
  line L34 (-2, 10.8) -> (-2, 13.2) projected
  line L35 (-2, 27.8) -> (-2, 30.2) projected
  line L36 (-2, 227.8) -> (-2, 230.2) projected
  line L37 (-2, 210.8) -> (-2, 213.2) projected
  line L38 (-2, 210.5) -> (-2, 223.0549) projected
  line L39 (-2, 223.0549) -> (-2, 230.5) projected
  line L40 (-2, 230.5) -> (-2, 217.9451) projected
  line L41 (-2, 217.9451) -> (-2, 210.5) projected
  line L42 (-2, 202.8) -> (-2, 205.2) projected
  line L43 (-2, 185.8) -> (-2, 188.2) projected
  line L44 (-2, 185.5) -> (-2, 198.0549) projected
  line L45 (-2, 198.0549) -> (-2, 205.5) projected
  line L46 (-2, 205.5) -> (-2, 192.9451) projected
  line L47 (-2, 192.9451) -> (-2, 185.5) projected
  line L48 (-2, 177.8) -> (-2, 180.2) projected
  line L49 (-2, 160.8) -> (-2, 163.2) projected
  line L50 (-2, 160.5) -> (-2, 173.0549) projected
  line L51 (-2, 173.0549) -> (-2, 180.5) projected
  line L52 (-2, 180.5) -> (-2, 167.9451) projected
  line L53 (-2, 167.9451) -> (-2, 160.5) projected
  line L54 (-2, 135.5) -> (-2, 148.0549) projected
  line L55 (-2, 148.0549) -> (-2, 155.5) projected
  line L56 (-2, 155.5) -> (-2, 142.9451) projected
  line L57 (-2, 142.9451) -> (-2, 135.5) projected
  line L58 (-2, 135.8) -> (-2, 138.2) projected
  line L59 (-2, 152.8) -> (-2, 155.2) projected
  line L60 (-2, 192) -> (-2, 199) projected
  line L61 (-2, 192) -> (-2, 199) projected
  line L62 (-2, 167) -> (-2, 174) projected
  line L63 (-2, 167) -> (-2, 174) projected
  line L64 (-2, 17) -> (-2, 24) projected
  line L65 (-2, 17) -> (-2, 24) projected
  line L66 (-2, 142) -> (-2, 149) projected
  line L67 (-2, 142) -> (-2, 149) projected
  line L68 (-2, 42) -> (-2, 49) projected
  line L69 (-2, 42) -> (-2, 49) projected
  line L70 (-2, 117) -> (-2, 124) projected
  line L71 (-2, 117) -> (-2, 124) projected
  line L72 (-2, 24) -> (-2, 17) projected
  line L73 (-2, 3) -> (-2, 17) projected
  line L74 (-2, 3) -> (-2, 238) projected
  line L75 (-2, 224) -> (-2, 238) projected
  line L76 (-2, 224) -> (-2, 217) projected
  line L77 (-2, 199) -> (-2, 217) projected
  line L78 (-2, 199) -> (-2, 192) projected
  line L79 (-2, 174) -> (-2, 192) projected
  line L80 (-2, 174) -> (-2, 167) projected
  line L81 (-2, 149) -> (-2, 167) projected
  line L82 (-2, 149) -> (-2, 142) projected
  line L83 (-2, 124) -> (-2, 142) projected
  line L84 (-2, 124) -> (-2, 117) projected
  line L85 (-2, 99) -> (-2, 117) projected
  line L86 (-2, 99) -> (-2, 92) projected
  line L87 (-2, 74) -> (-2, 92) projected
  line L88 (-2, 74) -> (-2, 67) projected
  line L89 (-2, 49) -> (-2, 67) projected
  line L90 (-2, 49) -> (-2, 42) projected
  line L91 (-2, 24) -> (-2, 42) projected
  line L92 (-2, 67) -> (-2, 74) projected
  line L93 (-2, 67) -> (-2, 74) projected
  line L94 (-2, 92) -> (-2, 99) projected
  line L95 (-2, 92) -> (-2, 99) projected
  line L96 (-5, 17) -> (-5, 24) projected
  line L97 (-5, 24) -> (-5, 17) projected
  line L98 (-5, 3) -> (-2, 3) projected
  line L99 (-5, 3) -> (-12, 3) projected
  line L100 (-2, 3) -> (-12, 3) projected
  line L101 (-2, 3) -> (-2, 238) projected
  line L102 (-5, 3) -> (-2, 3)
  line L103 (-2, 3) -> (-2, 238)
  line L104 (-2, 238) -> (-5, 238)
  line L105 (-5, 238) -> (-5, 3)
  point P0 (0, 120.5)
  point P1 (-5, 3)
  constraints: 8 end point, 2 parallel, 1 horizontal, 1 perpendicular
extrude "Vysunutí9" cut sketch "Náčrt9" against normal up to surface (3 mm away) contours L9 L8 L5 L74 L15 L12 L14 L13 L21 L18 L20 L19 L27 L24 L26 L25 L31 L30 L73 L98 L105 L96 L104 L39 L36 L6 L38 L37 L45 L42 L44 L43 L51 L48 L50 L49 L55 L54 L4
sketch "Náčrt10" plane through (0, 0, 2) normal (0, 0, 1) x (1, 0, 0)
  circle A0 centre (-15, 8.5) radius 1.2 projected
  circle A1 centre (15, -8.5) radius 1.2 projected
  line L0 (23.5, 96.5) -> (23.5, 103.5) projected
  line L1 (23.5, 96.5) -> (22, 96.5) projected
  line L2 (22, 96.5) -> (22, 103.5) projected
  line L3 (22, 103.5) -> (23.5, 103.5) projected
  line L4 (9.1905, -10) -> (-15.8095, -10) projected
  line L5 (-15.8095, -10) -> (-15.8095, 2.5549) projected
  arc A2 (-15.8095, 2.5549) -> (-9.1905, 10) centre (-15, 8.5) ccw projected
  line L6 (-9.1905, 10) -> (15.8095, 10) projected
  line L7 (15.8095, 10) -> (15.8095, -2.5549) projected
  arc A3 (15.8095, -2.5549) -> (9.1905, -10) centre (15, -8.5) ccw projected
  circle A4 centre (-15, -16.5) radius 1.2 projected
  circle A5 centre (15, -33.5) radius 1.2 projected
  line L8 (9.1905, -35) -> (-15.8095, -35) projected
  line L9 (-15.8095, -35) -> (-15.8095, -22.4451) projected
  arc A6 (-15.8095, -22.4451) -> (-9.1905, -15) centre (-15, -16.5) ccw projected
  line L10 (-9.1905, -15) -> (15.8095, -15) projected
  line L11 (15.8095, -15) -> (15.8095, -27.5549) projected
  arc A7 (15.8095, -27.5549) -> (9.1905, -35) centre (15, -33.5) ccw projected
  circle A8 centre (-15, -41.5) radius 1.2 projected
  circle A9 centre (15, -58.5) radius 1.2 projected
  line L12 (9.1905, -60) -> (-15.8095, -60) projected
  line L13 (-15.8095, -60) -> (-15.8095, -47.4451) projected
  arc A10 (-15.8095, -47.4451) -> (-9.1905, -40) centre (-15, -41.5) ccw projected
  line L14 (-9.1905, -40) -> (15.8095, -40) projected
  line L15 (15.8095, -40) -> (15.8095, -52.5549) projected
  arc A11 (15.8095, -52.5549) -> (9.1905, -60) centre (15, -58.5) ccw projected
  circle A12 centre (-15, -66.5) radius 1.2 projected
  circle A13 centre (15, -83.5) radius 1.2 projected
  line L16 (9.1905, -85) -> (-15.8095, -85) projected
  line L17 (-15.8095, -85) -> (-15.8095, -72.4451) projected
  arc A14 (-15.8095, -72.4451) -> (-9.1905, -65) centre (-15, -66.5) ccw projected
  line L18 (-9.1905, -65) -> (15.8095, -65) projected
  line L19 (15.8095, -65) -> (15.8095, -77.5549) projected
  arc A15 (15.8095, -77.5549) -> (9.1905, -85) centre (15, -83.5) ccw projected
  line L20 (9.1905, -110) -> (-15.8095, -110) projected
  line L21 (-15.8095, -110) -> (-15.8095, -97.4451) projected
  arc A16 (-15.8095, -97.4451) -> (-9.1905, -90) centre (-15, -91.5) ccw projected
  line L22 (-9.1905, -90) -> (15.8095, -90) projected
  line L23 (15.8095, -90) -> (15.8095, -102.5549) projected
  arc A17 (15.8095, -102.5549) -> (9.1905, -110) centre (15, -108.5) ccw projected
  circle A18 centre (15, -108.5) radius 1.2 projected
  circle A19 centre (-15, -91.5) radius 1.2 projected
  circle A20 centre (-15, 108.5) radius 1.2 projected
  circle A21 centre (15, 91.5) radius 1.2 projected
  line L24 (9.1905, 90) -> (-15.8095, 90) projected
  line L25 (-15.8095, 90) -> (-15.8095, 102.5549) projected
  arc A22 (-15.8095, 102.5549) -> (-9.1905, 110) centre (-15, 108.5) ccw projected
  line L26 (-9.1905, 110) -> (15.8095, 110) projected
  line L27 (15.8095, 110) -> (15.8095, 97.4451) projected
  arc A23 (15.8095, 97.4451) -> (9.1905, 90) centre (15, 91.5) ccw projected
  circle A24 centre (-15, 83.5) radius 1.2 projected
  circle A25 centre (15, 66.5) radius 1.2 projected
  line L28 (9.1905, 65) -> (-15.8095, 65) projected
  line L29 (-15.8095, 65) -> (-15.8095, 77.5549) projected
  arc A26 (-15.8095, 77.5549) -> (-9.1905, 85) centre (-15, 83.5) ccw projected
  line L30 (-9.1905, 85) -> (15.8095, 85) projected
  line L31 (15.8095, 85) -> (15.8095, 72.4451) projected
  arc A27 (15.8095, 72.4451) -> (9.1905, 65) centre (15, 66.5) ccw projected
  circle A28 centre (-15, 58.5) radius 1.2 projected
  circle A29 centre (15, 41.5) radius 1.2 projected
  line L32 (9.1905, 40) -> (-15.8095, 40) projected
  line L33 (-15.8095, 40) -> (-15.8095, 52.5549) projected
  arc A30 (-15.8095, 52.5549) -> (-9.1905, 60) centre (-15, 58.5) ccw projected
  line L34 (-9.1905, 60) -> (15.8095, 60) projected
  line L35 (15.8095, 60) -> (15.8095, 47.4451) projected
  arc A31 (15.8095, 47.4451) -> (9.1905, 40) centre (15, 41.5) ccw projected
  line L36 (9.1905, 15) -> (-15.8095, 15) projected
  line L37 (-15.8095, 15) -> (-15.8095, 27.5549) projected
  arc A32 (-15.8095, 27.5549) -> (-9.1905, 35) centre (-15, 33.5) ccw projected
  line L38 (-9.1905, 35) -> (15.8095, 35) projected
  line L39 (15.8095, 35) -> (15.8095, 22.4451) projected
  arc A33 (15.8095, 22.4451) -> (9.1905, 15) centre (15, 16.5) ccw projected
  circle A34 centre (15, 16.5) radius 1.2 projected
  circle A35 centre (-15, 33.5) radius 1.2 projected
  line L40 (23.5, 71.5) -> (22, 71.5) projected
  line L41 (22, 71.5) -> (22, 78.5) projected
  line L42 (22, 78.5) -> (23.5, 78.5) projected
  line L43 (23.5, 71.5) -> (23.5, 78.5) projected
  line L44 (23.5, 46.5) -> (22, 46.5) projected
  line L45 (22, 46.5) -> (22, 53.5) projected
  line L46 (22, 53.5) -> (23.5, 53.5) projected
  line L47 (23.5, 46.5) -> (23.5, 53.5) projected
  line L48 (23.5, -103.5) -> (23.5, -96.5) projected
  line L49 (23.5, -103.5) -> (22, -103.5) projected
  line L50 (22, -103.5) -> (22, -96.5) projected
  line L51 (22, -96.5) -> (23.5, -96.5) projected
  line L52 (23.5, 21.5) -> (22, 21.5) projected
  line L53 (22, 21.5) -> (22, 28.5) projected
  line L54 (22, 28.5) -> (23.5, 28.5) projected
  line L55 (23.5, 21.5) -> (23.5, 28.5) projected
  line L56 (23.5, -78.5) -> (23.5, -71.5) projected
  line L57 (23.5, -78.5) -> (22, -78.5) projected
  line L58 (22, -78.5) -> (22, -71.5) projected
  line L59 (22, -71.5) -> (23.5, -71.5) projected
  line L60 (23.5, -3.5) -> (22, -3.5) projected
  line L61 (22, -3.5) -> (22, 3.5) projected
  line L62 (22, 3.5) -> (23.5, 3.5) projected
  line L63 (23.5, -3.5) -> (23.5, 3.5) projected
  line L64 (-31.5, -96.5) -> (-22, -96.5) projected
  line L65 (-22, -96.5) -> (-22, -103.5) projected
  line L66 (-22, -103.5) -> (-31.5, -103.5) projected
  line L67 (-31.5, -117.5) -> (-31.5, -103.5) projected
  line L68 (-31.5, -117.5) -> (31.5, -117.5) projected
  line L69 (31.5, 117.5) -> (31.5, -117.5) projected
  line L70 (31.5, 117.5) -> (-31.5, 117.5) projected
  line L71 (-31.5, 103.5) -> (-31.5, 117.5) projected
  line L72 (-31.5, 103.5) -> (-22, 103.5) projected
  line L73 (-22, 103.5) -> (-22, 96.5) projected
  line L74 (-22, 96.5) -> (-31.5, 96.5) projected
  line L75 (-31.5, 78.5) -> (-31.5, 96.5) projected
  line L76 (-31.5, 78.5) -> (-22, 78.5) projected
  line L77 (-22, 78.5) -> (-22, 71.5) projected
  line L78 (-22, 71.5) -> (-31.5, 71.5) projected
  line L79 (-31.5, 53.5) -> (-31.5, 71.5) projected
  line L80 (-31.5, 53.5) -> (-22, 53.5) projected
  line L81 (-22, 53.5) -> (-22, 46.5) projected
  line L82 (-22, 46.5) -> (-31.5, 46.5) projected
  line L83 (-31.5, 28.5) -> (-31.5, 46.5) projected
  line L84 (-31.5, 28.5) -> (-22, 28.5) projected
  line L85 (-22, 28.5) -> (-22, 21.5) projected
  line L86 (-22, 21.5) -> (-31.5, 21.5) projected
  line L87 (-31.5, 3.5) -> (-31.5, 21.5) projected
  line L88 (-31.5, 3.5) -> (-22, 3.5) projected
  line L89 (-22, 3.5) -> (-22, -3.5) projected
  line L90 (-22, -3.5) -> (-31.5, -3.5) projected
  line L91 (-31.5, -21.5) -> (-31.5, -3.5) projected
  line L92 (-31.5, -21.5) -> (-22, -21.5) projected
  line L93 (-22, -21.5) -> (-22, -28.5) projected
  line L94 (-22, -28.5) -> (-31.5, -28.5) projected
  line L95 (-31.5, -46.5) -> (-31.5, -28.5) projected
  line L96 (-31.5, -46.5) -> (-22, -46.5) projected
  line L97 (-22, -46.5) -> (-22, -53.5) projected
  line L98 (-22, -53.5) -> (-31.5, -53.5) projected
  line L99 (-31.5, -71.5) -> (-31.5, -53.5) projected
  line L100 (-31.5, -71.5) -> (-22, -71.5) projected
  line L101 (-22, -71.5) -> (-22, -78.5) projected
  line L102 (-22, -78.5) -> (-31.5, -78.5) projected
  line L103 (-31.5, -96.5) -> (-31.5, -78.5) projected
  line L104 (23.5, -53.5) -> (23.5, -46.5) projected
  line L105 (23.5, -53.5) -> (22, -53.5) projected
  line L106 (22, -53.5) -> (22, -46.5) projected
  line L107 (22, -46.5) -> (23.5, -46.5) projected
  line L108 (23.5, -28.5) -> (22, -28.5) projected
  line L109 (22, -28.5) -> (22, -21.5) projected
  line L110 (22, -21.5) -> (23.5, -21.5) projected
  line L111 (23.5, -28.5) -> (23.5, -21.5) projected
  line L112 (23.5, 21.5) -> (23.5, 28.5) projected
  line L113 (23.5, 21.5) -> (31.5, 21.5)
  line L114 (31.5, 21.5) -> (31.5, 28.5)
  line L115 (31.5, 28.5) -> (23.5, 28.5)
  line L116 (23.5, 28.5) -> (23.5, 21.5)
  line L117 (23.5, 46.5) -> (22, 46.5) projected
  line L118 (23.5, 46.5) -> (31.5, 46.5)
  line L119 (31.5, 46.5) -> (31.5, 53.5)
  line L120 (31.5, 53.5) -> (23.5, 53.5)
  line L121 (23.5, 53.5) -> (23.5, 46.5)
  line L122 (23.5, 71.5) -> (23.5, 78.5) projected
  line L123 (23.5, 71.5) -> (31.5, 71.5)
  line L124 (31.5, 71.5) -> (31.5, 78.5)
  line L125 (31.5, 78.5) -> (23.5, 78.5)
  line L126 (23.5, 78.5) -> (23.5, 71.5)
  line L127 (23.5, 96.5) -> (31.5, 96.5)
  line L128 (31.5, 96.5) -> (31.5, 103.5)
  line L129 (31.5, 103.5) -> (23.5, 103.5)
  line L130 (23.5, 103.5) -> (23.5, 96.5)
  line L131 (23.5, -3.5) -> (31.5, -3.5)
  line L132 (31.5, -3.5) -> (31.5, 3.5)
  line L133 (31.5, 3.5) -> (23.5, 3.5)
  line L134 (23.5, 3.5) -> (23.5, -3.5)
  line L135 (23.5, -28.5) -> (31.5, -28.5)
  line L136 (31.5, -28.5) -> (31.5, -21.5)
  line L137 (31.5, -21.5) -> (23.5, -21.5)
  line L138 (23.5, -21.5) -> (23.5, -28.5)
  line L139 (23.5, -53.5) -> (22, -53.5) projected
  line L140 (23.5, -53.5) -> (31.5, -53.5)
  line L141 (31.5, -53.5) -> (31.5, -46.5)
  line L142 (31.5, -46.5) -> (23.5, -46.5)
  line L143 (23.5, -46.5) -> (23.5, -53.5)
  line L144 (23.5, -78.5) -> (31.5, -78.5)
  line L145 (31.5, -78.5) -> (31.5, -71.5)
  line L146 (31.5, -71.5) -> (23.5, -71.5)
  line L147 (23.5, -71.5) -> (23.5, -78.5)
  line L148 (23.5, -103.5) -> (31.5, -103.5)
  line L149 (31.5, -103.5) -> (31.5, -96.5)
  line L150 (31.5, -96.5) -> (23.5, -96.5)
  line L151 (23.5, -96.5) -> (23.5, -103.5)
  point P0 (0, 0)
  point P1 (31.5, 96.5)
  point P2 (31.5, 21.5)
  point P3 (31.5, -3.5)
  point P4 (31.5, -53.5)
  constraints: 72 end point, 18 parallel, 9 horizontal, 9 perpendicular, 9 point on line, 10 other
extrude "Vysunutí10" add sketch "Náčrt10" along normal up to surface (3 mm away) contours L0 L129 L69 L127 | L69 L123 L43 L125 | L69 L118 L47 L120 | L69 L113 L55 L115 | L69 L131 L63 L133 | L69 L135 L111 L137 | L69 L140 L104 L142 | L69 L144 L56 L146 | L69 L148 L48 L150
fillet "Zaoblení2" radius 1.5 4 edges at (31.5, 120.5, 6) (-31.5, 120.5, 6) (-31.5, -120.5, 6) (31.5, -120.5, 6)
fillet "Zaoblení4" radius 1 18 edges at (22, -100, 5) (-22, -100, 5) (-22, -75, 5) (22, -75, 5) (22, -50, 5) (-22, -50, 5) (22, -25, 5) (22, 0, 5) (22, 25, 5) (-22, 0, 5) (-22, -25, 5) (22, 50, 5) (-22, 25, 5) (-22, 50, 5) (-22, 75, 5) (22, 75, 5) (-22, 100, 5) (22, 100, 5)
sketch "Náčrt11" plane through (0, 0, 12) normal (0, 0, 1) x (1, 0, 0)
  arc A0 (30, -120.5) -> (31.5, -119) centre (30, -119) ccw projected
  line L0 (31.5, -119) -> (31.5, 119) projected
  arc A1 (31.5, 119) -> (30, 120.5) centre (30, 119) ccw projected
  line L1 (30, 120.5) -> (-30, 120.5) projected
  arc A2 (-30, 120.5) -> (-31.5, 119) centre (-30, 119) ccw projected
  line L2 (-31.5, 119) -> (-31.5, -119) projected
  arc A3 (-31.5, -119) -> (-30, -120.5) centre (-30, -119) ccw projected
  line L3 (-30, -120.5) -> (30, -120.5) projected
  line L4 (28.5, 117.5) -> (28.5, -117.5) projected
  line L5 (28.5, -117.5) -> (-28.5, -117.5) projected
  line L6 (-28.5, -117.5) -> (-28.5, 117.5) projected
  line L7 (-28.5, 117.5) -> (28.5, 117.5) projected
  line L8 (-31.5, -117.5) -> (-28.5, -117.5) projected
  line L9 (28.5, 117.5) -> (-28.5, 117.5)
  line L10 (-28.5, 117.5) -> (-28.5, -117.5)
  line L11 (-28.5, -117.5) -> (28.5, -117.5)
  line L12 (28.5, -117.5) -> (28.5, 117.5)
  line L13 (29.95, -118.95) -> (-29.95, -118.95)
  line L14 (-29.95, -118.95) -> (-29.95, 118.95)
  line L15 (-29.95, 118.95) -> (29.95, 118.95)
  line L16 (29.95, 118.95) -> (29.95, -118.95)
  point P0 (0, 0)
  dimension "d50" = 1.45
  constraints: 16 end point, 4 parallel, 2 perpendicular, 1 horizontal, 3 other
  measures "d50" distance between parallel lines of L11 L13
extrude "Vysunutí11" add sketch "Náčrt11" along normal blind 3 contours L13 L14 L15 L16
